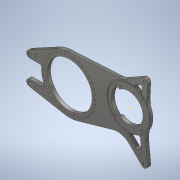
# Autodesk Inventor part: Plate
Saved by Autodesk Inventor 2021 (Build 250183000, 183)
## iProperties
Created: 2018-11-11
Part Number: Plate
Material: Stainless Steel, 440C
Document SubType Name: Modeling
Designer: steelen
Density: 7.75 g/cm^3
Appearance: Semi-Polished
Mass: 49446 g
Surface Area: 6759.07 cm^2
Volume: 6180.75 cm^3
Description: Left Mounting Plate
Material_size: 1/2" Aluminum Plate
Quantity: 1
Author: steelen
Autodesk Inventor part; units mm, degrees
ref_plane "YZ Plane" through (0, 0, 0) normal (1, 0, 0) x (0, 1, 0)
ref_plane "XZ Plane" through (0, 0, 0) normal (0, 1, 0) x (-1, 0, 0)
ref_plane "XY Plane" through (0, 0, 0) normal (0, 0, 1) x (1, 0, 0)
sketch "Sketch2" plane through (0, 0, 0) normal (0, 0, 1) x (1, 0, 0)
  circle A0 centre (0, 0) radius 82.55
  circle A1 centre (59.6616, 114.3) radius 12.7
  circle A2 centre (59.6616, -157.9372) radius 12.7
  line L0 (-9.194, 82.1469) -> (-13.3959, 81.4558)
  line L1 (-63.6408, 52.7493) -> (-60.758, 55.8835)
  circle A3 centre (-225.4026, -38.1) radius 107.95
  line L2 (53.382, 125.3389) -> (-40.8172, 71.7527)
  line L3 (72.3489, 113.732) -> (69.2676, 44.9055)
  line L4 (59.6616, 114.3) -> (0, 0)
  line L5 (0, 0) -> (59.6616, -157.9372)
  line L6 (72.2989, -156.6771) -> (62.0994, -54.389)
  line L7 (50.7023, -166.9384) -> (-58.2354, -58.5076)
  line L8 (-547.6025, 1708.7209) -> (-492.7385, 1708.7209)
  circle A4 centre (-377.8026, -107.1372) radius 12.7
  circle A5 centre (-377.8026, -12.7) radius 12.7
  line L9 (-377.8026, -25.4) -> (-332.603, -25.4)
  line L10 (-377.8026, -94.4372) -> (-317.4859, -94.4372)
  line L11 (59.6616, 114.3) -> (59.6616, -157.9372)
  line L12 (-380.0803, -119.6313) -> (-244.7629, -144.2997)
  line L13 (-383.8817, -1.5494) -> (-277.0748, 56.6797)
  point P0 (0, -82.55)
  point P1 (-24.2729, 78.9008)
  point P2 (0, -82.55)
  point P3 (-330.4145, -13.0858)
  point P4 (-67.641, 47.3201)
  point P5 (-322.3179, -85.6461)
  point P6 (55.5088, -61.1005)
  point P7 (-152.0839, -117.3311)
  point P8 (-49.767, -65.8616)
  point P9 (-69.6708, -44.2774)
  point P10 (-34.8418, 74.8368)
  point P11 (-213.235, 69.1621)
  point P12 (-270.3744, 60.0364)
  point P13 (-270.8002, -136.0401)
  dimension "d9" = 215.9
  dimension "d142" = 165.1
  dimension "d92" = 54.864
  dimension "d137" = 228.6
  dimension "d143" = 25.4
  dimension "d210" = 25.4
  dimension "d211" = 152.4
  dimension "d212" = 152.4
  dimension "d213" = 94.4372
  dimension "d214" = 25.4
  dimension "d235" = 272.2372
  dimension "d237" = 38.1
  dimension "d288" = 127
  dimension "d289" = 437.4642
  dimension "d302" = 25
  dimension "d303" = 15
  constraints: 28 end point, 8 point on circle, 8 tangent, 4 centre point, 3 horizontal, 2 equal radius, 1 coincident, 1 vertical, 34 other
  measures "d92" distance of L8.start L8.end
  measures "d137" distance of point (-225.403, -38.1) point (0, 0)
  measures "d143" diameter of A1
  measures "d210" diameter of A4
  measures "d211" horizontal distance of A4.centre point (-225.403, -38.1)
  measures "d212" horizontal distance of A5.centre point (-225.403, -38.1)
  measures "d213" distance of A4.centre A5.centre
  measures "d214" vertical distance of A5.centre point (-225.403, -38.1)
  measures "d235" distance of L4.start L5.end
  measures "d237" vertical distance of point (-225.403, -38.1) point (0, 0)
  measures "d288" vertical distance of L4.start A5.centre
  measures "d289" horizontal distance of L4.start A5.centre
  measures "d302" angle of L4 L3
  measures "d303" angle of L5 L6
extrude "Extrusion24" add sketch "Sketch2" along normal blind 12.7
sketch "Sketch35" plane through (0, 0, 12.7) normal (0, 0, 1) x (1, 0, 0)
  arc A0 (-332.603, -25.4) -> (-317.4859, -94.4372) centre (-225.4026, -38.1) ccw projected
  line L0 (-317.4859, -94.4372) -> (-377.8026, -94.4372) projected
  arc A1 (-377.8026, -94.4372) -> (-380.0803, -119.6313) centre (-377.8026, -107.1372) ccw projected
  arc A2 (-244.7629, -144.2997) -> (-277.0748, 56.6797) centre (-225.4026, -38.1) ccw projected
  arc A3 (-383.8817, -1.5494) -> (-377.8026, -25.4) centre (-377.8026, -12.7) ccw projected
  line L1 (-377.8026, -25.4) -> (-332.603, -25.4) projected
  circle A4 centre (-225.4026, -38.1) radius 85.725
  line L2 (-380.0803, -119.6313) -> (-244.7629, -144.2997) projected
  line L3 (-277.0748, 56.6797) -> (-383.8817, -1.5494) projected
  point P0 (0, 0)
  dimension "d266" = 171.45
  constraints: 1 centre point, 1 coincident
  measures "d266" diameter of A4
extrude "Extrusion28" cut sketch "Sketch35" against normal blind 12.7 contours A4
sketch "Sketch36" plane through (0, 0, 12.7) normal (0, 0, 1) x (1, 0, 0)
  arc A0 (-383.8817, -1.5494) -> (-377.8026, -25.4) centre (-377.8026, -12.7) ccw projected
  arc A1 (-377.8026, -94.4372) -> (-380.0803, -119.6313) centre (-377.8026, -107.1372) ccw projected
  arc A2 (72.3489, 113.732) -> (53.382, 125.3389) centre (59.6616, 114.3) ccw projected
  arc A3 (50.7023, -166.9384) -> (72.2989, -156.6771) centre (59.6616, -157.9372) ccw projected
  arc A4 (50.7023, -166.9384) -> (72.2989, -156.6771) centre (59.6616, -157.9372) ccw projected
  point P0 (0, 0)
  constraints: 4 coincident
hole "Hole9" at (-377.8026, -12.7, 12.7) at (-377.8026, -107.1372, 12.7) at (59.6616, 114.3, 12.7) at (59.6616, -157.9372, 12.7) direction (0, 0, -1) diameter 9.8044 depth 12.2936 tip angle 118 clearance for "Flat Head Machine Screw (82)" size "3/8" standard "Ansi Unified Screw Threads"
sketch "Sketch40" plane through (0, 0, 12.7) normal (0, 0, 1) x (1, 0, 0)
  circle A0 centre (-225.4026, -38.1) radius 85.725 projected
  line L0 (-225.4026, -136.525) -> (-225.4026, 60.325)
  line L1 (-323.8276, -38.1) -> (-126.9776, -38.1)
  point P0 (0, 0)
  point P1 (-150.0047, 25.1664)
  point P2 (-162.1363, -113.4979)
  point P3 (-300.8006, -101.3664)
  point P4 (-288.669, 37.2979)
  point P5 (-208.3113, 58.8297)
  point P6 (-128.4729, -55.1913)
  point P7 (-242.494, -135.0297)
  point P8 (-322.3323, -21.0087)
  point P9 (-274.6151, 47.1386)
  point P10 (-140.1641, 11.1125)
  point P11 (-176.1901, -123.3386)
  point P12 (-310.6412, -87.3125)
  point P13 (-317.8919, -4.4367)
  point P14 (-191.7393, 54.3892)
  point P15 (-132.9134, -71.7633)
  point P16 (-259.066, -130.5892)
  point P17 (-317.8919, -71.7633)
  point P18 (-259.066, 54.3892)
  point P19 (-132.9134, -4.4367)
  point P20 (-191.7393, -130.5892)
  point P21 (-274.6151, -123.3386)
  point P22 (-310.6412, 11.1125)
  point P23 (-176.1901, 47.1386)
  point P24 (-140.1641, -87.3125)
  point P25 (-208.3113, -135.0297)
  point P26 (-322.3323, -55.1913)
  point P27 (-242.494, 58.8297)
  point P28 (-128.4729, -21.0087)
  point P29 (-150.0047, -101.3664)
  point P30 (-288.669, -113.4979)
  point P31 (-300.8006, 25.1664)
  point P32 (-162.1363, 37.2979)
  dimension "d290" = 196.85
  dimension "d293" = 360
  constraints: 5 coincident, 4 end point, 2 midpoint, 1 horizontal, 1 perpendicular, 1 vertical, 37 other
  measures "d290" distance of L0.start L0.end
hole "Hole11" at (-225.4026, 60.325, 12.7) at (-225.4026, -136.525, 12.7) at (-323.8276, -38.1, 12.7) at (-126.9776, -38.1, 12.7) at (-150.0047, 25.1664, 12.7) at (-162.1363, -113.4979, 12.7) at (-300.8006, -101.3664, 12.7) at (-288.669, 37.2979, 12.7) at (-208.3113, 58.8297, 12.7) at (-128.4729, -55.1913, 12.7) at (-242.494, -135.0297, 12.7) at (-322.3323, -21.0087, 12.7) at (-274.6151, 47.1386, 12.7) at (-140.1641, 11.1125, 12.7) at (-176.1901, -123.3386, 12.7) at (-310.6412, -87.3125, 12.7) at (-317.8919, -4.4367, 12.7) at (-191.7393, 54.3892, 12.7) at (-132.9134, -71.7633, 12.7) at (-259.066, -130.5892, 12.7) at (-317.8919, -71.7633, 12.7) at (-259.066, 54.3892, 12.7) at (-132.9134, -4.4367, 12.7) at (-191.7393, -130.5892, 12.7) at (-274.6151, -123.3386, 12.7) at (-310.6412, 11.1125, 12.7) at (-176.1901, 47.1386, 12.7) at (-140.1641, -87.3125, 12.7) at (-208.3113, -135.0297, 12.7) at (-322.3323, -55.1913, 12.7) at (-242.494, 58.8297, 12.7) at (-128.4729, -21.0087, 12.7) at (-150.0047, -101.3664, 12.7) at (-288.669, -113.4979, 12.7) at (-300.8006, 25.1664, 12.7) at (-162.1363, 37.2979, 12.7) direction (0, 0, -1) diameter 6.5278 end through all clearance for "Socket Head Cap Screw" size "1/4" standard "Ansi Unified Screw Threads"
sketch "Sketch43" plane through (0, 0, 12.7) normal (0, 0, 1) x (1, 0, 0)
  circle A0 centre (-377.8026, -12.7) radius 4.9022 projected
  line L0 (-377.8026, -12.7) -> (-352.4026, -2.6443)
  line L1 (-277.0748, 56.6797) -> (-383.8817, -1.5494) projected
  circle A1 centre (-377.8026, -107.1372) radius 4.9022 projected
  line L2 (-377.8026, -107.1372) -> (-352.4026, -107.1372)
  circle A2 centre (59.6616, 114.3) radius 4.9022 projected
  line L3 (69.2676, 44.9055) -> (72.3489, 113.732) projected
  line L4 (53.382, 125.3389) -> (-40.8172, 71.7527) projected
  circle A3 centre (59.6616, -157.9372) radius 4.2258 projected
  line L5 (59.6616, -157.9372) -> (46.9616, -131.2079)
  line L6 (-58.2354, -58.5076) -> (50.7023, -166.9384) projected
  line L7 (72.2989, -156.6771) -> (62.0994, -54.389) projected
  point P0 (0, 0)
  point P1 (-23.9752, 81.3335)
  point P2 (-23.8818, -92.7013)
  dimension "d316" = 25.4
  dimension "d317" = 7
  dimension "d318" = 25.4
  dimension "d319" = 57.803
  dimension "d322" = 39.439
  dimension "d323" = 19.72
  dimension "d324" = 12.7
  constraints: 6 end point, 3 coincident, 1 horizontal
  measures "d316" horizontal distance of L0.start L0.end
  measures "d317" angle of L1 L0
  measures "d318" distance of L2.start L2.end
  measures "d319" angle of L3 L4
  measures "d322" angle of L6 L7
  measures "d323" angle of L7 L5
  measures "d324" horizontal distance of L5.start L5.end
hole "Hole13" at (-352.4026, -2.6443, 12.7) at (-352.4026, -107.1372, 12.7) at (46.9616, -131.2079, 12.7) direction (0, 0, -1) diameter 6.7564 end through all clearance for "Flat Head Machine Screw (82)" size "1/4" standard "Ansi Unified Screw Threads"
sketch "Sketch45" plane through (0, 0, 12.7) normal (0, 0, 1) x (1, 0, 0)
  arc A0 (40.4911, 64.5516) -> (-48.9804, 58.3726) centre (0, 0) ccw
  arc A1 (-48.9804, -58.3726) -> (40.4911, -64.5516) centre (0, 0) ccw
  circle A2 centre (0, 0) radius 63.5
  line L0 (-32.6536, -38.9151) -> (-48.9804, -58.3726)
  line L1 (40.4911, -64.5516) -> (26.9941, -43.0344)
  line L2 (30.4077, 48.4764) -> (40.4911, 64.5516)
  line L3 (-48.9804, 58.3726) -> (-32.6536, 38.9151)
  line L4 (0, 0) -> (0, -55.8244)
  line L5 (0, -55.8244) -> (-30.2636, -55.8244)
  line L6 (0, 59.4547) -> (0, 0)
  line L7 (0, 59.4547) -> (22.3022, 59.4547)
  point P0 (0, 0)
  point P1 (0, 0)
  point P2 (22.3022, -59.4547)
  point P3 (-30.2636, 55.8244)
  point P4 (25.4, -43.9941)
  point P5 (25.4, 43.9941)
  point P6 (26.9941, -43.0344)
  point P7 (30.4077, 48.4764)
  dimension "d332" = 12.7
  dimension "d333" = 12.7
  dimension "d334" = 12.7
  dimension "d335" = 12.7
  dimension "d336" = 12.7
  dimension "d337" = 76.2
  dimension "d338" = 127
  dimension "d381" = 30.2636
  dimension "d382" = 59.4547
  dimension "d383" = 22.3022
  dimension "d384" = 59.4547
  dimension "d429" = 49.025
  dimension "d430" = 22.3022
  dimension "d431" = 55.8244
  constraints: 12 end point, 8 point on circle, 3 centre point, 1 coincident, 1 horizontal, 1 perpendicular, 1 vertical, 6 other
  measures "d332" radial gap between concentric circles of A1 A2
  measures "d333" distance from line of L0 L5.end
  measures "d336" distance from line of L3 point (-30.264, 55.824)
  measures "d337" radius of A0
  measures "d338" diameter of A2
  measures "d381" distance of L4.end L5.end
  measures "d382" distance of L6.start L4.start
  measures "d383" distance of L6.start L7.end
  measures "d384" vertical distance of point (0, 0) A2.end
  measures "d430" horizontal distance of point (0, 0) A2.end
  measures "d431" vertical distance of L5.end point (0, 0)
hole "Hole14" at (-30.2636, -55.8244, 12.7) at (22.3022, -59.4547, 12.7) at (-30.2636, 55.8244, 12.7) at (22.3022, 59.4547, 12.7) direction (0, 0, -1) diameter 4.9784 end through all
sketch "Sketch46" plane through (0, 0, 12.7) normal (0, 0, 1) x (1, 0, 0)
  circle A0 centre (0, 0) radius 38.1
  dimension "d346" = 76.2
  constraints: 1 centre point, 1 coincident
  measures "d346" diameter of A0
extrude "Extrusion30" cut sketch "Sketch46" against normal blind 25.4
sketch "Sketch47" plane through (0, 0, 0) normal (0, 0, -1) x (-1, 0, 0)
  arc A0 (-69.2676, 44.9055) -> (-62.0994, -54.389) centre (0, 0) ccw projected
  arc A1 (58.2354, -58.5076) -> (-62.0994, -54.389) centre (0, 0) ccw projected
  line L0 (58.2354, -58.5076) -> (-50.7023, -166.9384) projected
  line L1 (-72.2989, -156.6771) -> (-62.0994, -54.389) projected
  line L2 (-69.2676, 44.9055) -> (-72.3489, 113.732) projected
  line L3 (-53.382, 125.3389) -> (40.8172, 71.7527) projected
  circle A2 centre (0, 0) radius 82.55
  line L4 (7.4118, -82.2166) -> (-26.473, -115.9437)
  arc A3 (-48.0696, -105.6824) -> (-26.473, -115.9437) centre (-35.4323, -106.9425) ccw
  line L5 (-48.0696, -105.6824) -> (-44.4667, -69.5501)
  line L6 (-51.0909, 64.84) -> (-52.289, 91.6024)
  line L7 (-42.8056, 97.4058) -> (-14.45, 81.2754)
  arc A4 (-42.8056, 97.4058) -> (-52.289, 91.6024) centre (-45.9454, 91.8864) ccw
  point P0 (62.6794, 53.7196)
  point P1 (23.8818, -92.7013)
  point P2 (23.9752, 81.3335)
  dimension "d349" = 19.05
  dimension "d350" = 19.05
  dimension "d351" = 12.7
  dimension "d353" = 19.05
  dimension "d354" = 19.05
  dimension "d355" = 6.35
  constraints: 8 end point, 8 point on circle, 4 parallel, 4 tangent, 3 centre point, 1 coincident, 1 concentric
  measures "d349" distance between parallel lines of L0 L4
  measures "d350" distance between parallel lines of L1 L5
  measures "d351" radius of A3
  measures "d353" distance between parallel lines of L2 L6
  measures "d354" distance between parallel lines of L3 L7
  measures "d355" radius of A4
extrude "Extrusion31" cut sketch "Sketch47" against normal blind 25.4 contours L6 A4 L7 A1 | A2 L4 A3 L5
sketch "Sketch48" plane through (0, 0, 0) normal (0, 0, -1) x (-1, 0, 0)
  line L0 (-52.289, 91.6024) -> (-51.0909, 64.84) projected
  arc A0 (-14.45, 81.2754) -> (-51.0909, 64.84) centre (0, 0) ccw projected
  line L1 (-14.45, 81.2754) -> (-42.8056, 97.4058) projected
  arc A1 (-42.8056, 97.4058) -> (-52.289, 91.6024) centre (-45.9454, 91.8864) ccw projected
  line L2 (-26.473, -115.9437) -> (7.4118, -82.2166) projected
  arc A2 (-44.4667, -69.5501) -> (7.4118, -82.2166) centre (0, 0) ccw projected
  line L3 (-44.4667, -69.5501) -> (-48.0696, -105.6824) projected
  arc A3 (-48.0696, -105.6824) -> (-26.473, -115.9437) centre (-35.4323, -106.9425) ccw projected
  circle A4 centre (0, 0) radius 38.1 projected
  circle A5 centre (30.2636, 55.8244) radius 2.4892 projected
  circle A6 centre (30.2636, -55.8244) radius 2.4892 projected
  circle A7 centre (-22.3022, -59.4547) radius 2.4892 projected
  circle A8 centre (-22.3022, 59.4547) radius 2.4892 projected
  circle A9 centre (352.4026, -107.1372) radius 3.3782 projected
  circle A10 centre (352.4026, -2.6443) radius 3.3782 projected
  circle A11 centre (-46.9616, -131.2079) radius 3.3782 projected
  circle A12 centre (300.8006, 25.1664) radius 3.2639 projected
  circle A13 centre (150.0047, -101.3664) radius 3.2639 projected
  circle A14 centre (242.494, 58.8297) radius 3.2639 projected
  circle A15 centre (208.3113, -135.0297) radius 3.2639 projected
  circle A16 centre (176.1901, 47.1386) radius 3.2639 projected
  circle A17 centre (274.6151, -123.3386) radius 3.2639 projected
  circle A18 centre (132.9134, -4.4367) radius 3.2639 projected
  circle A19 centre (317.8919, -71.7633) radius 3.2639 projected
  circle A20 centre (132.9134, -71.7633) radius 3.2639 projected
  circle A21 centre (317.8919, -4.4367) radius 3.2639 projected
  circle A22 centre (176.1901, -123.3386) radius 3.2639 projected
  circle A23 centre (274.6151, 47.1386) radius 3.2639 projected
  circle A24 centre (242.494, -135.0297) radius 3.2639 projected
  circle A25 centre (208.3113, 58.8297) radius 3.2639 projected
  circle A26 centre (300.8006, -101.3664) radius 3.2639 projected
  circle A27 centre (150.0047, 25.1664) radius 3.2639 projected
  circle A28 centre (323.8276, -38.1) radius 3.2639 projected
  circle A29 centre (225.4026, 60.325) radius 3.2639 projected
  circle A30 centre (225.4026, -136.525) radius 3.2639 projected
  circle A31 centre (126.9776, -38.1) radius 3.2639 projected
  circle A32 centre (162.1363, -113.4979) radius 3.2639 projected
  circle A33 centre (288.669, 37.2979) radius 3.2639 projected
  circle A34 centre (128.4729, -55.1913) radius 3.2639 projected
  circle A35 centre (322.3323, -21.0087) radius 3.2639 projected
  circle A36 centre (140.1641, 11.1125) radius 3.2639 projected
  circle A37 centre (310.6412, -87.3125) radius 3.2639 projected
  circle A38 centre (191.7393, 54.3892) radius 3.2639 projected
  circle A39 centre (259.066, -130.5892) radius 3.2639 projected
  circle A40 centre (259.066, 54.3892) radius 3.2639 projected
  circle A41 centre (191.7393, -130.5892) radius 3.2639 projected
  circle A42 centre (310.6412, 11.1125) radius 3.2639 projected
  circle A43 centre (140.1641, -87.3125) radius 3.2639 projected
  circle A44 centre (322.3323, -55.1913) radius 3.2639 projected
  circle A45 centre (128.4729, -21.0087) radius 3.2639 projected
  circle A46 centre (288.669, -113.4979) radius 3.2639 projected
  circle A47 centre (162.1363, 37.2979) radius 3.2639 projected
  circle A48 centre (377.8026, -12.7) radius 4.2258 projected
  circle A49 centre (377.8026, -107.1372) radius 4.2258 projected
  circle A50 centre (225.4026, -38.1) radius 85.725 projected
  circle A51 centre (-59.6616, 114.3) radius 4.2258 projected
  circle A52 centre (-59.6616, -157.9372) radius 4.2258 projected
  arc A53 (-69.2676, 44.9055) -> (-62.0994, -54.389) centre (0, 0) ccw projected
  line L4 (-69.2676, 44.9055) -> (-72.3489, 113.732) projected
  arc A54 (-53.382, 125.3389) -> (-72.3489, 113.732) centre (-59.6616, 114.3) ccw projected
  line L5 (-53.382, 125.3389) -> (40.8172, 71.7527) projected
  line L6 (277.0748, 56.6797) -> (383.8817, -1.5494) projected
  arc A55 (377.8026, -25.4) -> (383.8817, -1.5494) centre (377.8026, -12.7) ccw projected
  line L7 (377.8026, -25.4) -> (332.603, -25.4) projected
  line L8 (317.4859, -94.4372) -> (377.8026, -94.4372) projected
  arc A56 (380.0803, -119.6313) -> (377.8026, -94.4372) centre (377.8026, -107.1372) ccw projected
  line L9 (380.0803, -119.6313) -> (244.7629, -144.2997) projected
  line L10 (58.2354, -58.5076) -> (-50.7023, -166.9384) projected
  arc A57 (-72.2989, -156.6771) -> (-50.7023, -166.9384) centre (-59.6616, -157.9372) ccw projected
  line L11 (-72.2989, -156.6771) -> (-62.0994, -54.389) projected
  arc A58 (317.4859, -94.4372) -> (332.603, -25.4) centre (225.4026, -38.1) ccw projected
  arc A59 (322.482, -85.3101) -> (328.1926, -94.4372) centre (328.1926, -88.0872) ccw
  line L12 (377.8026, -25.4) -> (332.603, -25.4) projected
  arc A60 (339.5261, -25.4) -> (333.1859, -32.1028) centre (339.5261, -31.75) ccw
  arc A61 (-44.4667, -69.5501) -> (7.4118, -82.2166) centre (0, 0) ccw projected
  arc A62 (-3.467, -93.0447) -> (-7.379, -82.2195) centre (-7.9466, -88.5441) ccw
  arc A63 (-36.3171, -74.1321) -> (-45.4294, -79.2045) centre (-39.1107, -79.8346) ccw
  arc A64 (-14.45, 81.2754) -> (-51.0909, 64.84) centre (0, 0) ccw projected
  line L13 (-14.45, 81.2754) -> (-42.8056, 97.4058) projected
  arc A65 (-28.7219, 77.3922) -> (-27.7915, 88.8649) centre (-30.9313, 83.3454) ccw
  line L14 (-51.0909, 64.84) -> (-52.289, 91.6024) projected
  arc A66 (-51.601, 76.2338) -> (-42.0247, 71.0523) centre (-45.2574, 76.5178) ccw
  line L15 (-48.0696, -105.6824) -> (-44.4667, -69.5501) projected
  line L16 (7.4118, -82.2166) -> (-26.473, -115.9437) projected
  arc A67 (317.4859, -94.4372) -> (332.603, -25.4) centre (225.4026, -38.1) ccw projected
  arc A68 (128.2435, -85.1457) -> (135.8106, -98.3201) centre (225.4026, -38.1) ccw
  arc A69 (277.0748, 56.6797) -> (244.7629, -144.2997) centre (225.4026, -38.1) ccw projected
  arc A70 (317.4859, -94.4372) -> (332.603, -25.4) centre (225.4026, -38.1) ccw projected
  arc A71 (58.2354, -58.5076) -> (40.8172, 71.7527) centre (0, 0) ccw projected
  line L17 (317.4859, -94.4372) -> (377.8026, -94.4372) projected
  point P0 (160.5805, 48.2209)
  dimension "d358" = 6.35
  constraints: 19 point on circle, 14 tangent, 7 centre point, 6 point on line, 5 equal radius
  measures "d358" radius of A59
extrude "Extrusion32" add sketch "Sketch48" against normal up to surface (12.7 mm away) contours A66 A0 L0 | L1 A0 A65 | A62 A2 L2 | L3 A2 A63 | A60 A58 L7 | A59 L8 A58
sketch "Sketch49" plane through (0, 0, 0) normal (0, 0, -1) x (-1, 0, 0)
  arc A0 (-28.7219, 77.3922) -> (-27.7915, 88.8649) centre (-30.9313, 83.3454) ccw projected
  line L0 (-27.7915, 88.8649) -> (-42.8056, 97.4058) projected
  arc A1 (-42.8056, 97.4058) -> (-52.289, 91.6024) centre (-45.9454, 91.8864) ccw projected
  line L1 (-52.289, 91.6024) -> (-51.601, 76.2338) projected
  arc A2 (-51.601, 76.2338) -> (-42.0247, 71.0523) centre (-45.2574, 76.5178) ccw projected
  arc A3 (-28.7219, 77.3922) -> (-42.0247, 71.0523) centre (0, 0) ccw projected
  arc A4 (-36.3171, -74.1321) -> (-45.4294, -79.2045) centre (-39.1107, -79.8346) ccw projected
  line L2 (-45.4294, -79.2045) -> (-48.0696, -105.6824) projected
  arc A5 (-48.0696, -105.6824) -> (-26.473, -115.9437) centre (-35.4323, -106.9425) ccw projected
  line L3 (-26.473, -115.9437) -> (-3.467, -93.0447) projected
  arc A6 (-3.467, -93.0447) -> (-7.379, -82.2195) centre (-7.9466, -88.5441) ccw projected
  arc A7 (-36.3171, -74.1321) -> (-7.379, -82.2195) centre (0, 0) ccw projected
  circle A8 centre (0, 0) radius 38.1 projected
  circle A9 centre (30.2636, 55.8244) radius 2.4892 projected
  circle A10 centre (30.2636, -55.8244) radius 2.4892 projected
  circle A11 centre (-22.3022, -59.4547) radius 2.4892 projected
  circle A12 centre (-22.3022, 59.4547) radius 2.4892 projected
  circle A13 centre (-46.9616, -131.2079) radius 3.3782 projected
  circle A14 centre (-59.6616, 114.3) radius 4.2258 projected
  circle A15 centre (-59.6616, -157.9372) radius 4.2258 projected
  arc A16 (58.2354, -58.5076) -> (40.8172, 71.7527) centre (0, 0) ccw projected
  line L4 (58.2354, -58.5076) -> (-50.7023, -166.9384) projected
  arc A17 (-72.2989, -156.6771) -> (-50.7023, -166.9384) centre (-59.6616, -157.9372) ccw projected
  line L5 (-72.2989, -156.6771) -> (-62.0994, -54.389) projected
  arc A18 (-69.2676, 44.9055) -> (-62.0994, -54.389) centre (0, 0) ccw projected
  line L6 (-69.2676, 44.9055) -> (-72.3489, 113.732) projected
  arc A19 (-53.382, 125.3389) -> (-72.3489, 113.732) centre (-59.6616, 114.3) ccw projected
  line L7 (-53.382, 125.3389) -> (40.8172, 71.7527) projected
  circle A20 centre (352.4026, -107.1372) radius 3.3782 projected
  circle A21 centre (352.4026, -2.6443) radius 3.3782 projected
  circle A22 centre (300.8006, 25.1664) radius 3.2639 projected
  circle A23 centre (150.0047, -101.3664) radius 3.2639 projected
  circle A24 centre (242.494, 58.8297) radius 3.2639 projected
  circle A25 centre (208.3113, -135.0297) radius 3.2639 projected
  circle A26 centre (176.1901, 47.1386) radius 3.2639 projected
  circle A27 centre (274.6151, -123.3386) radius 3.2639 projected
  circle A28 centre (132.9134, -4.4367) radius 3.2639 projected
  circle A29 centre (317.8919, -71.7633) radius 3.2639 projected
  circle A30 centre (132.9134, -71.7633) radius 3.2639 projected
  circle A31 centre (317.8919, -4.4367) radius 3.2639 projected
  circle A32 centre (176.1901, -123.3386) radius 3.2639 projected
  circle A33 centre (274.6151, 47.1386) radius 3.2639 projected
  circle A34 centre (242.494, -135.0297) radius 3.2639 projected
  circle A35 centre (208.3113, 58.8297) radius 3.2639 projected
  circle A36 centre (300.8006, -101.3664) radius 3.2639 projected
  circle A37 centre (150.0047, 25.1664) radius 3.2639 projected
  circle A38 centre (323.8276, -38.1) radius 3.2639 projected
  circle A39 centre (225.4026, 60.325) radius 3.2639 projected
  circle A40 centre (225.4026, -136.525) radius 3.2639 projected
  circle A41 centre (126.9776, -38.1) radius 3.2639 projected
  circle A42 centre (162.1363, -113.4979) radius 3.2639 projected
  circle A43 centre (288.669, 37.2979) radius 3.2639 projected
  circle A44 centre (128.4729, -55.1913) radius 3.2639 projected
  circle A45 centre (322.3323, -21.0087) radius 3.2639 projected
  circle A46 centre (140.1641, 11.1125) radius 3.2639 projected
  circle A47 centre (310.6412, -87.3125) radius 3.2639 projected
  circle A48 centre (191.7393, 54.3892) radius 3.2639 projected
  circle A49 centre (259.066, -130.5892) radius 3.2639 projected
  circle A50 centre (259.066, 54.3892) radius 3.2639 projected
  circle A51 centre (191.7393, -130.5892) radius 3.2639 projected
  circle A52 centre (310.6412, 11.1125) radius 3.2639 projected
  circle A53 centre (140.1641, -87.3125) radius 3.2639 projected
  circle A54 centre (322.3323, -55.1913) radius 3.2639 projected
  circle A55 centre (128.4729, -21.0087) radius 3.2639 projected
  circle A56 centre (288.669, -113.4979) radius 3.2639 projected
  circle A57 centre (162.1363, 37.2979) radius 3.2639 projected
  circle A58 centre (377.8026, -12.7) radius 4.2258 projected
  circle A59 centre (377.8026, -107.1372) radius 4.2258 projected
  circle A60 centre (225.4026, -38.1) radius 85.725 projected
  arc A61 (277.0748, 56.6797) -> (244.7629, -144.2997) centre (225.4026, -38.1) ccw projected
  line L8 (277.0748, 56.6797) -> (383.8817, -1.5494) projected
  arc A62 (377.8026, -25.4) -> (383.8817, -1.5494) centre (377.8026, -12.7) ccw projected
  line L9 (377.8026, -25.4) -> (339.5261, -25.4) projected
  arc A63 (339.5261, -25.4) -> (333.1859, -32.1028) centre (339.5261, -31.75) ccw projected
  arc A64 (322.482, -85.3101) -> (333.1859, -32.1028) centre (225.4026, -38.1) ccw projected
  arc A65 (322.482, -85.3101) -> (328.1926, -94.4372) centre (328.1926, -88.0872) ccw projected
  line L10 (328.1926, -94.4372) -> (377.8026, -94.4372) projected
  arc A66 (380.0803, -119.6313) -> (377.8026, -94.4372) centre (377.8026, -107.1372) ccw projected
  line L11 (380.0803, -119.6313) -> (244.7629, -144.2997) projected
  arc A67 (277.0748, 56.6797) -> (244.7629, -144.2997) centre (225.4026, -38.1) ccw projected
  line L12 (231.4562, 69.6801) -> (23.9752, 81.3335)
  arc A68 (58.2354, -58.5076) -> (40.8172, 71.7527) centre (0, 0) ccw projected
  line L13 (195.6957, -141.882) -> (23.8818, -92.7013)
  line L14 (58.2354, -58.5076) -> (-50.7023, -166.9384) projected
  arc A69 (-36.3171, -74.1321) -> (-7.379, -82.2195) centre (0, 0) ccw projected
  arc A70 (-28.7219, 77.3922) -> (-42.0247, 71.0523) centre (0, 0) ccw projected
  line L15 (-53.382, 125.3389) -> (40.8172, 71.7527) projected
  line L16 (120.7808, -94.018) -> (54.894, -75.1583)
  line L17 (144.9717, 49.0976) -> (76.046, 52.9689)
  arc A71 (120.7808, -94.018) -> (128.2435, -85.1457) centre (122.5282, -87.9131) ccw
  arc A72 (149.1038, 38.2655) -> (144.9717, 49.0976) centre (144.6156, 42.7576) ccw
  arc A73 (76.046, 52.9689) -> (70.2835, 43.2982) centre (75.6899, 46.6289) ccw
  arc A74 (277.0748, 56.6797) -> (244.7629, -144.2997) centre (225.4026, -38.1) ccw projected
  arc A75 (58.2354, -58.5076) -> (40.8172, 71.7527) centre (0, 0) ccw projected
  line L18 (23.9752, 81.3335) -> (40.8172, 71.7527)
  line L19 (-53.382, 125.3389) -> (40.8172, 71.7527) projected
  arc A76 (231.4562, 69.6801) -> (149.1038, 38.2655) centre (225.4026, -38.1) ccw
  arc A77 (70.2835, 43.2982) -> (40.8172, 71.7527) centre (0, 0) ccw
  arc A78 (52.1619, -64.5529) -> (54.894, -75.1583) centre (56.6415, -69.0535) ccw
  line L20 (58.2354, -58.5076) -> (-50.7023, -166.9384) projected
  line L21 (52.1619, -64.5529) -> (23.8818, -92.7013)
  arc A79 (128.2435, -85.1457) -> (195.6957, -141.882) centre (225.4026, -38.1) ccw
  dimension "d361" = 25.4
  dimension "d362" = 25.4
  dimension "d363" = 6.35
  constraints: 19 point on circle, 14 tangent, 12 end point, 7 centre point, 3 point on line, 2 collinear, 2 equal radius, 2 parallel, 7 other
  measures "d361" distance between parallel lines of L12 L17
  measures "d362" distance between parallel lines of L13 L16
  measures "d363" radius of A71
extrude "Extrusion33" add sketch "Sketch49" against normal up to surface (12.7 mm away) contours A16 L7 L12 A61 A72 L17 A73 | A78 L16 A71 A61 L13 L4
sketch "Sketch50" plane through (0, 0, 12.7) normal (0, 0, 1) x (1, 0, 0)
  line L0 (-23.8818, -92.7013) -> (50.7023, -166.9384) projected
  line L1 (-23.8818, -92.7013) -> (-195.6957, -141.882) projected
  arc A0 (2.544, -119.0042) -> (-59.7271, -102.9618) centre (-42.2525, -164.0101) ccw
  line L2 (-231.4562, 69.6801) -> (-23.9752, 81.3335) projected
  arc A1 (-38.8567, 80.4977) -> (-11.0197, 88.7033) centre (-42.4176, 143.8978) ccw
  line L3 (69.2676, 44.9055) -> (72.3489, 113.732) projected
  arc A2 (62.0994, -54.389) -> (69.2676, 44.9055) centre (0, 0) ccw projected
  arc A3 (70.0386, 62.1276) -> (75.4424, 33.5104) centre (133.475, 59.2876) ccw
  line L4 (72.2989, -156.6771) -> (62.0994, -54.389) projected
  arc A4 (72.1103, -40.1821) -> (64.3931, -77.392) centre (127.5798, -71.0915) ccw
  line L5 (53.382, 125.3389) -> (-23.9752, 81.3335) projected
  arc A5 (62.0994, -54.389) -> (69.2676, 44.9055) centre (0, 0) ccw projected
  dimension "d366" = 63.5
  constraints: 10 point on circle, 8 tangent, 6 point on line, 4 centre point, 3 equal radius
  measures "d366" radius of A1
extrude "Extrusion34" add sketch "Sketch50" against normal up to surface (12.7 mm away)
chamfer "Chamfer2" distance 0.3969 angle 45 8 edges at (-377.8026, -102.235, 12.7) (-377.8026, -7.7978, 12.7) (59.6616, -153.035, 12.7) (59.6616, 119.2022, 12.7) (-377.8026, -8.4742, 0) (-377.8026, -102.9114, 0) (59.6616, -153.7114, 0) (59.6616, 118.5258, 0)
sketch "Sketch53" plane through (0, 0, 12.7) normal (0, 0, 1) x (1, 0, 0)
  circle A0 centre (0, 0) radius 84.455
  circle A1 centre (0, 0) radius 79.375
  dimension "d376" = 168.91
  dimension "d377" = 158.75
  constraints: 2 centre point, 2 coincident
  measures "d376" diameter of A0
  measures "d377" diameter of A1
extrude "Extrusion35" cut sketch "Sketch53" against normal blind 1.905
sketch "Sketch55" plane through (0, 0, 12.7) normal (0, 0, 1) x (1, 0, 0)
  arc A0 (-70.2835, 43.2982) -> (-58.2354, -58.5076) centre (0, 0) ccw projected
  arc A1 (-43.6177, -49.9541) -> (-31.8117, -32.9899) centre (-43.7741, -37.255) ccw
  arc A2 (-31.8117, 32.9899) -> (-46.3835, 47.3971) centre (-44.3737, 34.8572) ccw
  arc A3 (-31.8117, 32.9899) -> (-31.8117, -32.9899) centre (0, 0) ccw
  arc A4 (-46.3835, 47.3971) -> (-43.6177, -49.9541) centre (0, 0) ccw
  dimension "d395" = 12.7
  dimension "d396" = 12.7
  constraints: 8 point on circle, 4 centre point, 2 coincident
  measures "d395" radius of A1
  measures "d396" radius of A2
extrude "Extrusion37" cut sketch "Sketch55" against normal blind 25.4
sketch "Sketch57" plane through (0, 0, 12.7) normal (0, 0, 1) x (1, 0, 0)
  circle A0 centre (0, 0) radius 38.1 projected
  arc A1 (-21.5789, 50.8309) -> (-13.0971, 28.4028) centre (-13.4196, 41.0987) ccw
  arc A2 (13.0702, 28.4152) -> (13.6296, 53.5132) centre (11.4179, 41.0073) ccw
  arc A3 (13.0702, 28.4152) -> (-13.0971, 28.4028) centre (0, 0) ccw
  arc A4 (13.6296, 53.5132) -> (-21.5789, 50.8309) centre (0, 0) ccw
  dimension "d405" = 12.7
  dimension "d406" = 12.7
  constraints: 8 point on circle, 4 centre point, 2 coincident
  measures "d405" radius of A1
  measures "d406" radius of A2
extrude "Extrusion39" cut sketch "Sketch57" against normal blind 25.4
sketch "Sketch58" plane through (0, 0, 12.7) normal (0, 0, 1) x (1, 0, 0)
  point P0 (0, 0)
sketch "Sketch59" plane through (0, 0, 0) normal (0, 0, -1) x (-1, 0, 0)
  point P0 (0, 0)
  point P1 (-51.054, 51.054)
  point P2 (-51.054, -51.054)
  point P3 (51.054, -51.054)
  point P4 (51.054, 51.054)
  dimension "d407" = 51.054
  dimension "d408" = 51.054
  dimension "d409" = 51.054
  dimension "d410" = 51.054
  dimension "d411" = 51.054
  dimension "d412" = 51.054
  dimension "d413" = 51.054
  dimension "d414" = 51.054
  measures "d407" horizontal distance of point (0, 0) point (-51.054, 51.054)
  measures "d408" horizontal distance of point (0, 0) point (-51.054, 51.054)
  measures "d409" horizontal distance of point (0, 0) point (51.054, 51.054)
  measures "d410" horizontal distance of point (0, 0) point (51.054, 51.054)
  measures "d411" horizontal distance of point (0, 0) point (51.054, -51.054)
  measures "d412" horizontal distance of point (51.054, -51.054) point (0, 0)
  measures "d413" horizontal distance of point (0, 0) point (-51.054, -51.054)
  measures "d414" horizontal distance of point (0, 0) point (-51.054, -51.054)
hole "Hole15" at (51.054, 51.054, 0) at (51.054, -51.054, 0) at (-51.054, -51.054, 0) at (-51.054, 51.054, 0) direction (0, 0, 1) diameter 4.9784 end through all thread size "1/4-20 UNC" class "2B" standard "ANSI Unified Screw Threads"
sketch "Sketch60" plane through (0, 0, 0) normal (0, 0, -1) x (-1, 0, 0)
  circle A0 centre (0, 0) radius 76.5683
  arc A1 (-20.4908, 32.1207) -> (21.6008, 31.3849) centre (0, 0) ccw projected
  circle A2 centre (0, 0) radius 84.201
  dimension "d422" = 153.1366
  dimension "d423" = 168.402
  constraints: 2 centre point, 2 coincident
  measures "d422" diameter of A0
  measures "d423" diameter of A2
extrude "Extrusion40" cut sketch "Sketch60" against normal blind 1.905
sketch "Sketch62" plane through (0, 0, 0) normal (0, 0, -1) x (-1, 0, 0)
  circle A0 centre (0, 0) radius 55.4401
  constraints: 1 centre point, 1 coincident
extrude "Extrusion41" cut sketch "Sketch62" against normal blind 25.4
fillet "Fillet2" radius 3.175 2 edges at (-34.7773, 43.1758, 6.35) (-33.2496, -44.363, 6.35)
sketch "Sketch63" plane through (0, 0, 12.7) normal (0, 0, 1) x (1, 0, 0)
  arc A0 (-70.2835, 43.2982) -> (-69.4894, 47.9987) centre (-75.6899, 46.6289) ccw projected
  arc A1 (-69.4894, 47.9987) -> (-76.046, 52.9689) centre (-75.6899, 46.6289) ccw projected
  line L0 (-76.046, 52.9689) -> (-144.9717, 49.0976) projected
  arc A2 (-70.2835, 43.2982) -> (-58.2354, -58.5076) centre (0, 0) ccw projected
  line L1 (-52.1619, -64.5529) -> (-58.2354, -58.5076) projected
  arc A3 (-54.894, -75.1583) -> (-50.4272, -67.7476) centre (-56.6415, -69.0535) ccw projected
  arc A4 (-50.4272, -67.7476) -> (-52.1619, -64.5529) centre (-56.6415, -69.0535) ccw projected
  line L2 (-120.7808, -94.018) -> (-54.894, -75.1583) projected
  arc A5 (-128.2435, -85.1457) -> (-120.7808, -94.018) centre (-122.5282, -87.9131) ccw projected
  arc A6 (-128.2435, -85.1457) -> (-149.1038, 38.2655) centre (-225.4026, -38.1) ccw projected
  arc A7 (-144.9717, 49.0976) -> (-149.1038, 38.2655) centre (-144.6156, 42.7576) ccw projected
extrude "Extrusion42" add sketch "Sketch63" against normal up to surface (12.7 mm away)
equation "\"Angle\" = 12deg"
body "Solid2"
